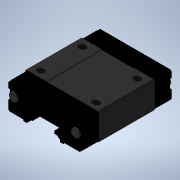
# Autodesk Inventor part: SSEB-MX13_b
Saved by Autodesk Inventor 2021 (Build 250183000, 183)
## iProperties
Created: 2025-02-22
Part Number: SSEB-MX13_b
Material: Generic
Catalog Web Link: www.cadenas.de
Description: SSEB, SSEB-MX, SSEBV, SSEBV-MX, SSE2B, SSE2B-MX, SSE2BV, SSE2BV-MX, SSEBL, SSEBL-MX, SSEBLV, SSEBLV-MX, SSE2BL, SSE2BL-MX, SSE2BLV, SSE2BLV-MX, SEB, SEBV, SE2B, SE2BV, SEBL, SEBLV, SE2BL, SE2BLV_block-Miniature Linear Guides - Short Block, Standard Preload - High/Precision Grade
Vendor: MISUMI
Document SubType Name: Modeling
Designer: psAdmin
Manufacturer: MISUMI
Mass: 6.93419 g
Surface Area: 35.9078 cm^2
Volume: 6.93419 cm^3
Density: 1 g/cm^3
Appearance: PSOLRGB-175-175-175
Category: PARTsolutions
Company: MISUMI
Title: SSEB-MX13
Author: Cadenas PARTsolutions
Comments: Miniature Linear Guides - Short Block, Standard Preload - High/Precision Grade
PSOL_IDENT_0: {$CADENAS_DATA/23d-libs/misumi/metric/06_linear_guides/seb_series/seb_block.prj},367 {VTYP=3D},{NB=S
PSOL_IDENT_1: SEB-MX13_b},{LINA=SSEB-MX13},{NN=SSEB, SSEB-MX, SSEBV, SSEBV-MX, SSE2B, SSE2B-MX, SSE2BV, SSE2BV-MX,
PSOL_IDENT_2: SSEBL, SSEBL-MX, SSEBLV, SSEBLV-MX, SSE2BL, SSE2BL-MX, SSE2BLV, SSE2BLV-MX, SEB, SEBV, SE2B, SE2BV,
PSOL_IDENT_3: SEBL, SEBLV, SE2BL, SE2BLV_block},{DATE=01.06.2021 05:33:03},{GEOMDATE=29.09.2020 01:45:00},{VERSIO
PSOL_IDENT_4: N=},{LINEID=230},{WBVAR=TS,MAT,ST,MX},{WBNUMERIC=}  {NB=SSEB-MX13_b},{LINA=SSEB-MX13},{KT=DUMMY},{PN=
PSOL_IDENT_5: SSEB-MX13},{TS=},{TYPE=SSEB},{H=13},{MAT=S},{ST=S},{ST1='S', 'w/o Surface Treatment','R','Low Temper
PSOL_IDENT_6: ature Black Chrome Plating'},{HARD=56HRC~},{STPN=S},{MX=-MX},{MXALG='', 'w/o MX(Lubrication unit)', '
PSOL_IDENT_7: -MX', 'with MX(Lubrication unit)'},{W=27},{L1=33.9},{B=20},{C=15},{SLL=M3x3.5},{S=3},{LL=3.5},{L2=19
PSOL_IDENT_8: .9},{K=10.0},{CBB=0.5},{W1=12},{W2=7.5},{H1=7.5},{CAA=0.5},{F=25},{G=10.0},{CA1=0.3},{CA2=0.5},{VA1=
PSOL_IDENT_9: 2.3},{HA1=2.0},{WA1=2.5298},{WA2=1.0},{RA1=2.64},{HA2=12.5830},{POIA1=0.1820},{BHA1=22.6},{BHA2=26.5
PSOL_IDENT_10: },{BHA3=26.6},{BHA5=15.0000},{BHA6=26.1},{BHA7=10.8},{BHA8=3.2},{BVA1=4.60},{BVA3=0.30},{BVA4=0.40},
PSOL_IDENT_11: {BVA5=9.50},{BVA6=9.60},{BCA1=0.5},{BCA2H=0.4},{BCA2V=0.25},{BRA1=1.80},{BRA2=1.50},{BDA1=24.00},{BH
PSOL_IDENT_12: B1=14.4600},{BHB2=12.9382},{BVB1=5.6300},{BVB2=2.6106},{BRB1=1.6},{BRB2=1.3000},{BRB3=0.1},{BHC1=5.5
PSOL_IDENT_13: 0},{BHC2=1.0},{BHC3=0.6},{BHC4=0.4},{BHC5=0.5},{MD=6.5}
NB: SSEB-MX13_b
NN: SSEB, SSEB-MX, SSEBV, SSEBV-MX, SSE2B, SSE2B-MX, SSE2BV, SSE2BV-MX, SSEBL, SSEBL-MX, SSEBLV, SSEBLV-MX, SSE2BL, SSE2BL-MX, SSE2BLV, SSE2BLV-MX, SEB, SEBV, SE2B, SE2BV, SEBL, SEBLV, SE2BL, SE2BLV_block
NT: Miniature Linear Guides - Short Block, Standard Preload - High/Precision Grade
NBSYN: $PN._b
LINA: SSEB-MX13
CATALOG: Misumi
PN: SSEB-MX13
TS: Advanced
H: 13
MAT: Stainless Steel
ST: w/o Surface Treatment
MX: with MX(Lubrication unit)
W: 27
L1: 33.9
B: 20
C: 15
SLL: M3x3.5
S: 3
LL: 3.5
L2: 19.9
K: 10
CBB: 0.5
W1: 12
W2: 7.5
H1: 7.5
CAA: 0.5
F: 25
G: 10
CA1: 0.3
CA2: 0.5
VA1: 2.3
HA1: 2
WA1: 2.5298
WA2: 1
RA1: 2.64
HA2: 12.583
POIA1: 0.182
BHA1: 22.6
BHA2: 26.5
BHA3: 26.6
BHA5: 15
BHA6: 26.1
BHA7: 10.8
BHA8: 3.2
BVA1: 4.6
BVA3: 0.3
BVA4: 0.4
BVA5: 9.5
BVA6: 9.6
BCA1: 0.5
BCA2H: 0.4
BCA2V: 0.25
BRA1: 1.8
BRA2: 1.5
BDA1: 24
BHB1: 14.46
BHB2: 12.9382
BVB1: 5.63
BVB2: 2.6106
BRB1: 1.6
BRB2: 1.3
BRB3: 0.1
BHC1: 5.5
BHC2: 1
BHC3: 0.6
BHC4: 0.4
BHC5: 0.5
MD: 6.5
SUPPLIER: MISUMI
ARTICLENO: SSEB-MX13_b
BOMINFO: SSEB-MX13
CREATOR: CADENAS GmbH
Autodesk Inventor part; units mm, degrees
sketch "Sketch_2" plane through (0, 0, 0) normal (0, 0, 1) x (1, 0, 0)
  line L0 (-13.5, 3.5) -> (-13, 3)
  line L1 (-13, 3) -> (-7.5, 3)
  line L2 (-7.5, 3) -> (-7.2754, 3.1)
  line L3 (-7.2754, 3.1) -> (7.2754, 3.1)
  line L4 (7.2754, 3.1) -> (7.5, 3)
  line L5 (7.5, 3) -> (13, 3)
  line L6 (13, 3) -> (13.5, 3.5)
  line L7 (13.5, 3.5) -> (13.5, 12.5)
  line L8 (13.5, 12.5) -> (13, 13)
  line L9 (13, 13) -> (5.8, 13)
  line L10 (5.8, 13) -> (5.4, 12.75)
  line L11 (5.4, 12.75) -> (-5.4, 12.75)
  line L12 (-5.4, 12.75) -> (-5.8, 13)
  line L13 (-5.8, 13) -> (-13, 13)
  line L14 (-13, 13) -> (-13.5, 12.5)
  line L15 (-13.5, 12.5) -> (-13.5, 3.5)
  constraints: 32 end point
extrude "Extrusion1" add sketch "Sketch_2" along normal mid plane 19.9
sketch "Sketch_3" plane through (0, 0, 9.95) normal (0, 0, 1) x (1, 0, 0)
  line L0 (-13.3, 12.2) -> (-13.3, 3.6)
  line L1 (-13.3, 3.6) -> (-12.8, 3.1)
  line L2 (-12.8, 3.1) -> (12.8, 3.1)
  line L3 (12.8, 3.1) -> (13.3, 3.6)
  line L4 (13.3, 3.6) -> (13.3, 12.2)
  line L5 (13.3, 12.2) -> (12.8, 12.7)
  line L6 (12.8, 12.7) -> (-12.8, 12.7)
  line L7 (-12.8, 12.7) -> (-13.3, 12.2)
  constraints: 16 end point
extrude "Extrusion2" add sketch "Sketch_3" along normal blind 7
sketch "Sketch_4" plane through (0, 0, -9.95) normal (0, 0, 1) x (1, 0, 0)
  line L0 (-13.3, 12.2) -> (-13.3, 3.6)
  line L1 (-13.3, 3.6) -> (-12.8, 3.1)
  line L2 (-12.8, 3.1) -> (12.8, 3.1)
  line L3 (12.8, 3.1) -> (13.3, 3.6)
  line L4 (13.3, 3.6) -> (13.3, 12.2)
  line L5 (13.3, 12.2) -> (12.8, 12.7)
  line L6 (12.8, 12.7) -> (-12.8, 12.7)
  line L7 (-12.8, 12.7) -> (-13.3, 12.2)
  constraints: 16 end point
extrude "Extrusion3" add sketch "Sketch_4" against normal blind 7
sketch "Sketch_8" plane through (0, 0, 16.95) normal (0, 0, 1) x (1, 0, 0)
  line L0 (-27, 19.5) -> (-27, 0)
  line L1 (-27, 0) -> (27, 0)
  line L2 (27, 0) -> (27, 19.5)
  line L3 (27, 19.5) -> (-27, 19.5)
  line L4 (-13.25, 12.1) -> (-13.25, 10.2)
  line L5 (-13.25, 10.2) -> (-11.3, 10.2)
  arc A0 (-11.3, 6.6) -> (-11.3, 10.2) centre (-11.3, 8.4) ccw
  line L6 (-11.3, 6.6) -> (-13.25, 6.6)
  line L7 (-13.25, 6.6) -> (-13.25, 3.6)
  line L8 (-13.25, 3.6) -> (-12.75, 3.1)
  line L9 (-12.75, 3.1) -> (12.75, 3.1)
  line L10 (12.75, 3.1) -> (13.25, 3.6)
  line L11 (13.25, 3.6) -> (13.25, 6.6)
  line L12 (13.25, 6.6) -> (11.3, 6.6)
  arc A1 (11.3, 10.2) -> (11.3, 6.6) centre (11.3, 8.4) ccw
  line L13 (11.3, 10.2) -> (13.25, 10.2)
  line L14 (13.25, 10.2) -> (13.25, 12.1)
  line L15 (13.25, 12.1) -> (12.75, 12.6)
  line L16 (12.75, 12.6) -> (-12.75, 12.6)
  line L17 (-12.75, 12.6) -> (-13.25, 12.1)
  constraints: 36 end point, 4 point on circle, 2 centre point
extrude "Extrusion4" cut sketch "Sketch_8" against normal blind 1.5
sketch "Sketch_14" plane through (0, 0, 16.95) normal (0, 0, 1) x (1, 0, 0)
  line L0 (-27, 19.5) -> (-27, 0)
  line L1 (-27, 0) -> (27, 0)
  line L2 (27, 0) -> (27, 19.5)
  line L3 (27, 19.5) -> (-27, 19.5)
  arc A0 (-7.23, 6.5053) -> (-6.4, 5.2932) centre (-5.93, 6.5053) ccw
  arc A1 (-6.4, 5.1068) -> (-6.4, 5.2932) centre (-6.4362, 5.2) ccw
  arc A2 (-6.4, 5.1068) -> (-7.23, 3.8947) centre (-5.93, 3.8947) ccw
  line L4 (-7.23, 3.8947) -> (-7.23, 3.1)
  line L5 (-7.23, 3.1) -> (7.23, 3.1)
  line L6 (7.23, 3.1) -> (7.23, 3.8947)
  arc A3 (7.23, 3.8947) -> (6.4, 5.1068) centre (5.93, 3.8947) ccw
  arc A4 (6.4, 5.2932) -> (6.4, 5.1068) centre (6.4362, 5.2) ccw
  arc A5 (6.4, 5.2932) -> (7.23, 6.5053) centre (5.93, 6.5053) ccw
  line L7 (7.23, 6.5053) -> (7.23, 7.13)
  arc A6 (7.23, 7.13) -> (5.63, 8.73) centre (5.63, 7.13) ccw
  line L8 (5.63, 8.73) -> (-5.63, 8.73)
  arc A7 (-5.63, 8.73) -> (-7.23, 7.13) centre (-5.63, 7.13) ccw
  line L9 (-7.23, 7.13) -> (-7.23, 6.5053)
  constraints: 20 end point, 16 point on circle, 8 centre point
extrude "Extrusion5" cut sketch "Sketch_14" against normal blind 0.5
sketch "Sketch_7" plane through (0, 0, -16.95) normal (0, 0, 1) x (1, 0, 0)
  line L0 (-27, 19.5) -> (-27, 0)
  line L1 (-27, 0) -> (27, 0)
  line L2 (27, 0) -> (27, 19.5)
  line L3 (27, 19.5) -> (-27, 19.5)
  line L4 (-13.25, 12.1) -> (-13.25, 10.2)
  line L5 (-13.25, 10.2) -> (-11.3, 10.2)
  arc A0 (-11.3, 6.6) -> (-11.3, 10.2) centre (-11.3, 8.4) ccw
  line L6 (-11.3, 6.6) -> (-13.25, 6.6)
  line L7 (-13.25, 6.6) -> (-13.25, 3.6)
  line L8 (-13.25, 3.6) -> (-12.75, 3.1)
  line L9 (-12.75, 3.1) -> (12.75, 3.1)
  line L10 (12.75, 3.1) -> (13.25, 3.6)
  line L11 (13.25, 3.6) -> (13.25, 6.6)
  line L12 (13.25, 6.6) -> (11.3, 6.6)
  arc A1 (11.3, 10.2) -> (11.3, 6.6) centre (11.3, 8.4) ccw
  line L13 (11.3, 10.2) -> (13.25, 10.2)
  line L14 (13.25, 10.2) -> (13.25, 12.1)
  line L15 (13.25, 12.1) -> (12.75, 12.6)
  line L16 (12.75, 12.6) -> (-12.75, 12.6)
  line L17 (-12.75, 12.6) -> (-13.25, 12.1)
  constraints: 36 end point, 4 point on circle, 2 centre point
extrude "Extrusion6" cut sketch "Sketch_7" along normal blind 1.5
sketch "Sketch_16" plane through (0, 0, -16.95) normal (0, 0, 1) x (1, 0, 0)
  line L0 (-27, 19.5) -> (-27, 0)
  line L1 (-27, 0) -> (27, 0)
  line L2 (27, 0) -> (27, 19.5)
  line L3 (27, 19.5) -> (-27, 19.5)
  arc A0 (-7.23, 6.5053) -> (-6.4, 5.2932) centre (-5.93, 6.5053) ccw
  arc A1 (-6.4, 5.1068) -> (-6.4, 5.2932) centre (-6.4362, 5.2) ccw
  arc A2 (-6.4, 5.1068) -> (-7.23, 3.8947) centre (-5.93, 3.8947) ccw
  line L4 (-7.23, 3.8947) -> (-7.23, 3.1)
  line L5 (-7.23, 3.1) -> (7.23, 3.1)
  line L6 (7.23, 3.1) -> (7.23, 3.8947)
  arc A3 (7.23, 3.8947) -> (6.4, 5.1068) centre (5.93, 3.8947) ccw
  arc A4 (6.4, 5.2932) -> (6.4, 5.1068) centre (6.4362, 5.2) ccw
  arc A5 (6.4, 5.2932) -> (7.23, 6.5053) centre (5.93, 6.5053) ccw
  line L7 (7.23, 6.5053) -> (7.23, 7.13)
  arc A6 (7.23, 7.13) -> (5.63, 8.73) centre (5.63, 7.13) ccw
  line L8 (5.63, 8.73) -> (-5.63, 8.73)
  arc A7 (-5.63, 8.73) -> (-7.23, 7.13) centre (-5.63, 7.13) ccw
  line L9 (-7.23, 7.13) -> (-7.23, 6.5053)
  constraints: 20 end point, 16 point on circle, 8 centre point
extrude "Extrusion7" cut sketch "Sketch_16" along normal blind 0.5
sketch "Sketch_25" plane through (0, 0, 15.45) normal (0, 0, 1) x (1, 0, 0)
  line L0 (-13.05, 10.2) -> (-13.05, 6.6)
  line L1 (-13.05, 6.6) -> (-11.3, 6.6)
  arc A0 (-11.3, 6.6) -> (-11.3, 10.2) centre (-11.3, 8.4) ccw
  line L2 (-11.3, 10.2) -> (-13.05, 10.2)
  constraints: 6 end point, 2 point on circle, 1 centre point
extrude "Extrusion8" add sketch "Sketch_25" along normal blind 0.6
sketch "Sketch_5" plane through (0, 0, 15.45) normal (0, 0, 1) x (1, 0, 0)
  arc A0 (11.3, 10.2) -> (11.3, 6.6) centre (11.3, 8.4) ccw
  line L0 (11.3, 6.6) -> (13.05, 6.6)
  line L1 (13.05, 6.6) -> (13.05, 10.2)
  line L2 (13.05, 10.2) -> (11.3, 10.2)
  constraints: 6 end point, 2 point on circle, 1 centre point
extrude "Extrusion9" add sketch "Sketch_5" along normal blind 0.6
sketch "Sketch_9" plane through (0, 0, -15.45) normal (0, 0, 1) x (1, 0, 0)
  line L0 (-13.05, 10.2) -> (-13.05, 6.6)
  line L1 (-13.05, 6.6) -> (-11.3, 6.6)
  arc A0 (-11.3, 6.6) -> (-11.3, 10.2) centre (-11.3, 8.4) ccw
  line L2 (-11.3, 10.2) -> (-13.05, 10.2)
  constraints: 6 end point, 2 point on circle, 1 centre point
extrude "Extrusion10" add sketch "Sketch_9" against normal blind 0.6
sketch "Sketch_26" plane through (0, 0, -15.45) normal (0, 0, 1) x (1, 0, 0)
  arc A0 (11.3, 10.2) -> (11.3, 6.6) centre (11.3, 8.4) ccw
  line L0 (11.3, 6.6) -> (13.05, 6.6)
  line L1 (13.05, 6.6) -> (13.05, 10.2)
  line L2 (13.05, 10.2) -> (11.3, 10.2)
  constraints: 6 end point, 2 point on circle, 1 centre point
extrude "Extrusion11" add sketch "Sketch_26" against normal blind 0.6
sketch "Sketch_18" plane through (-11.3, 0, 0) normal (1, 0, 0) x (0, 0, -1)
  line L0 (-16.05, 8.4) -> (-16.65, 8.4)
  line L1 (-16.65, 8.4) -> (-16.65, 9.9)
  line L2 (-16.65, 9.9) -> (-16.05, 9.9)
  line L3 (-16.05, 9.9) -> (-16.05, 8.4)
  line L4 (-16.05, 8.4) -> (-16.65, 8.4)
  constraints: 10 end point
revolve "Revolution1" add sketch "Sketch_18" angle 360 about axis through (-11.3, 8.4, 16.05) along (0, 0, -1)
sketch "Sketch_19" plane through (-11.3, 0, 0) normal (1, 0, 0) x (0, 0, -1)
  line L0 (16.65, 8.4) -> (16.05, 8.4)
  line L1 (16.05, 8.4) -> (16.05, 9.9)
  line L2 (16.05, 9.9) -> (16.65, 9.9)
  line L3 (16.65, 9.9) -> (16.65, 8.4)
  line L4 (16.65, 8.4) -> (16.05, 8.4)
  constraints: 10 end point
revolve "Revolution2" add sketch "Sketch_19" angle 360 about axis through (-11.3, 8.4, -16.65) along (0, 0, -1)
sketch "Sketch_20" plane through (11.3, 0, 0) normal (1, 0, 0) x (0, 0, -1)
  line L0 (-16.05, 8.4) -> (-16.65, 8.4)
  line L1 (-16.65, 8.4) -> (-16.65, 9.9)
  line L2 (-16.65, 9.9) -> (-16.05, 9.9)
  line L3 (-16.05, 9.9) -> (-16.05, 8.4)
  line L4 (-16.05, 8.4) -> (-16.65, 8.4)
  constraints: 10 end point
revolve "Revolution3" add sketch "Sketch_20" angle 360 about axis through (11.3, 8.4, 16.05) along (0, 0, -1)
sketch "Sketch_21" plane through (11.3, 0, 0) normal (1, 0, 0) x (0, 0, -1)
  line L0 (16.65, 8.4) -> (16.05, 8.4)
  line L1 (16.05, 8.4) -> (16.05, 9.9)
  line L2 (16.05, 9.9) -> (16.65, 9.9)
  line L3 (16.65, 9.9) -> (16.65, 8.4)
  line L4 (16.65, 8.4) -> (16.05, 8.4)
  constraints: 10 end point
revolve "Revolution4" add sketch "Sketch_21" angle 360 about axis through (11.3, 8.4, -16.65) along (0, 0, -1)
sketch "Sketch_17" plane through (0, 0, 0) normal (0, 0, 1) x (1, 0, 0)
  line L0 (-6, 7.2) -> (-6, 6.4649)
  line L1 (-6, 6.4649) -> (-5.6315, 6.2522)
  arc A0 (-5.1112, 5.7) -> (-5.6315, 6.2522) centre (-6.2915, 5.109) ccw
  line L2 (-5.1112, 5.7) -> (-4, 5.7)
  line L3 (-4, 5.7) -> (-4, 4.7)
  line L4 (-4, 4.7) -> (-5.1112, 4.7)
  arc A1 (-5.6315, 4.1478) -> (-5.1112, 4.7) centre (-6.2915, 5.291) ccw
  line L5 (-5.6315, 4.1478) -> (-6, 3.9351)
  line L6 (-6, 3.9351) -> (-6, 0.5)
  line L7 (-6, 0.5) -> (-5.5, 0)
  line L8 (-5.5, 0) -> (5.5, 0)
  line L9 (5.5, 0) -> (6, 0.5)
  line L10 (6, 0.5) -> (6, 3.9351)
  line L11 (6, 3.9351) -> (5.6315, 4.1478)
  arc A2 (5.1112, 4.7) -> (5.6315, 4.1478) centre (6.2915, 5.291) ccw
  line L12 (5.1112, 4.7) -> (4, 4.7)
  line L13 (4, 4.7) -> (4, 5.7)
  line L14 (4, 5.7) -> (5.1112, 5.7)
  arc A3 (5.6315, 6.2522) -> (5.1112, 5.7) centre (6.2915, 5.109) ccw
  line L15 (5.6315, 6.2522) -> (6, 6.4649)
  line L16 (6, 6.4649) -> (6, 7.2)
  line L17 (6, 7.2) -> (5.7, 7.5)
  line L18 (5.7, 7.5) -> (-5.7, 7.5)
  line L19 (-5.7, 7.5) -> (-6, 7.2)
  constraints: 40 end point, 8 point on circle, 4 centre point
extrude "Extrusion12" cut sketch "Sketch_17" along normal mid plane 19.9
sketch "Sketch_11" plane through (0, 0, 9.95) normal (0, 0, 1) x (1, 0, 0)
  line L0 (-6, 7.2) -> (-6, 6.4649)
  line L1 (-6, 6.4649) -> (-5.6315, 6.2522)
  arc A0 (-5.1112, 5.7) -> (-5.6315, 6.2522) centre (-6.2915, 5.109) ccw
  line L2 (-5.1112, 5.7) -> (-4, 5.7)
  line L3 (-4, 5.7) -> (-4, 4.7)
  line L4 (-4, 4.7) -> (-5.1112, 4.7)
  arc A1 (-5.6315, 4.1478) -> (-5.1112, 4.7) centre (-6.2915, 5.291) ccw
  line L5 (-5.6315, 4.1478) -> (-6, 3.9351)
  line L6 (-6, 3.9351) -> (-6, 0.5)
  line L7 (-6, 0.5) -> (-5.5, 0)
  line L8 (-5.5, 0) -> (5.5, 0)
  line L9 (5.5, 0) -> (6, 0.5)
  line L10 (6, 0.5) -> (6, 3.9351)
  line L11 (6, 3.9351) -> (5.6315, 4.1478)
  arc A2 (5.1112, 4.7) -> (5.6315, 4.1478) centre (6.2915, 5.291) ccw
  line L12 (5.1112, 4.7) -> (4, 4.7)
  line L13 (4, 4.7) -> (4, 5.7)
  line L14 (4, 5.7) -> (5.1112, 5.7)
  arc A3 (5.6315, 6.2522) -> (5.1112, 5.7) centre (6.2915, 5.109) ccw
  line L15 (5.6315, 6.2522) -> (6, 6.4649)
  line L16 (6, 6.4649) -> (6, 7.2)
  line L17 (6, 7.2) -> (5.7, 7.5)
  line L18 (5.7, 7.5) -> (-5.7, 7.5)
  line L19 (-5.7, 7.5) -> (-6, 7.2)
  constraints: 40 end point, 8 point on circle, 4 centre point
extrude "Extrusion13" cut sketch "Sketch_11" along normal blind 9.95
sketch "Sketch_22" plane through (0, 0, 9.95) normal (0, 0, 1) x (1, 0, 0)
  line L0 (-27, 19.5) -> (-27, 0)
  line L1 (-27, 0) -> (27, 0)
  line L2 (27, 0) -> (27, 19.5)
  line L3 (27, 19.5) -> (-27, 19.5)
  line L4 (-13.3, 12.25) -> (-13.3, 3.6)
  line L5 (-13.3, 3.6) -> (-12.85, 3.15)
  line L6 (-12.85, 3.15) -> (-6.05, 3.15)
  line L7 (-6.05, 3.15) -> (-6.05, 3.9851)
  line L8 (-6.05, 3.9851) -> (-5.7055, 4.1643)
  arc A0 (-5.7055, 4.1643) -> (-5.1425, 4.75) centre (-6.2915, 5.291) ccw
  line L9 (-5.1425, 4.75) -> (-4.05, 4.75)
  line L10 (-4.05, 4.75) -> (-4.05, 5.65)
  line L11 (-4.05, 5.65) -> (-5.1425, 5.65)
  arc A1 (-5.1425, 5.65) -> (-5.7055, 6.2357) centre (-6.2915, 5.109) ccw
  line L12 (-5.7055, 6.2357) -> (-6.05, 6.4149)
  line L13 (-6.05, 6.4149) -> (-6.05, 7.25)
  line L14 (-6.05, 7.25) -> (-5.75, 7.55)
  line L15 (-5.75, 7.55) -> (5.75, 7.55)
  line L16 (5.75, 7.55) -> (6.05, 7.25)
  line L17 (6.05, 7.25) -> (6.05, 6.4149)
  line L18 (6.05, 6.4149) -> (5.7055, 6.2357)
  arc A2 (5.7055, 6.2357) -> (5.1425, 5.65) centre (6.2915, 5.109) ccw
  line L19 (5.1425, 5.65) -> (4.05, 5.65)
  line L20 (4.05, 5.65) -> (4.05, 4.75)
  line L21 (4.05, 4.75) -> (5.1425, 4.75)
  arc A3 (5.1425, 4.75) -> (5.7055, 4.1643) centre (6.2915, 5.291) ccw
  line L22 (5.7055, 4.1643) -> (6.05, 3.9851)
  line L23 (6.05, 3.9851) -> (6.05, 3.15)
  line L24 (6.05, 3.15) -> (12.85, 3.15)
  line L25 (12.85, 3.15) -> (13.3, 3.6)
  line L26 (13.3, 3.6) -> (13.3, 12.25)
  line L27 (13.3, 12.25) -> (12.85, 12.7)
  line L28 (12.85, 12.7) -> (-12.85, 12.7)
  line L29 (-12.85, 12.7) -> (-13.3, 12.25)
  constraints: 60 end point, 8 point on circle, 4 centre point
extrude "Extrusion14" cut sketch "Sketch_22" along normal blind 0.05
sketch "Sketch_10" plane through (0, 0, -9.95) normal (0, 0, 1) x (1, 0, 0)
  line L0 (-6, 7.2) -> (-6, 6.4649)
  line L1 (-6, 6.4649) -> (-5.6315, 6.2522)
  arc A0 (-5.1112, 5.7) -> (-5.6315, 6.2522) centre (-6.2915, 5.109) ccw
  line L2 (-5.1112, 5.7) -> (-4, 5.7)
  line L3 (-4, 5.7) -> (-4, 4.7)
  line L4 (-4, 4.7) -> (-5.1112, 4.7)
  arc A1 (-5.6315, 4.1478) -> (-5.1112, 4.7) centre (-6.2915, 5.291) ccw
  line L5 (-5.6315, 4.1478) -> (-6, 3.9351)
  line L6 (-6, 3.9351) -> (-6, 0.5)
  line L7 (-6, 0.5) -> (-5.5, 0)
  line L8 (-5.5, 0) -> (5.5, 0)
  line L9 (5.5, 0) -> (6, 0.5)
  line L10 (6, 0.5) -> (6, 3.9351)
  line L11 (6, 3.9351) -> (5.6315, 4.1478)
  arc A2 (5.1112, 4.7) -> (5.6315, 4.1478) centre (6.2915, 5.291) ccw
  line L12 (5.1112, 4.7) -> (4, 4.7)
  line L13 (4, 4.7) -> (4, 5.7)
  line L14 (4, 5.7) -> (5.1112, 5.7)
  arc A3 (5.6315, 6.2522) -> (5.1112, 5.7) centre (6.2915, 5.109) ccw
  line L15 (5.6315, 6.2522) -> (6, 6.4649)
  line L16 (6, 6.4649) -> (6, 7.2)
  line L17 (6, 7.2) -> (5.7, 7.5)
  line L18 (5.7, 7.5) -> (-5.7, 7.5)
  line L19 (-5.7, 7.5) -> (-6, 7.2)
  constraints: 40 end point, 8 point on circle, 4 centre point
extrude "Extrusion15" cut sketch "Sketch_10" against normal blind 9.95
sketch "Sketch_23" plane through (0, 0, -9.95) normal (0, 0, 1) x (1, 0, 0)
  line L0 (-27, 19.5) -> (-27, 0)
  line L1 (-27, 0) -> (27, 0)
  line L2 (27, 0) -> (27, 19.5)
  line L3 (27, 19.5) -> (-27, 19.5)
  line L4 (-13.3, 12.25) -> (-13.3, 3.6)
  line L5 (-13.3, 3.6) -> (-12.85, 3.15)
  line L6 (-12.85, 3.15) -> (-6.05, 3.15)
  line L7 (-6.05, 3.15) -> (-6.05, 3.9851)
  line L8 (-6.05, 3.9851) -> (-5.7055, 4.1643)
  arc A0 (-5.7055, 4.1643) -> (-5.1425, 4.75) centre (-6.2915, 5.291) ccw
  line L9 (-5.1425, 4.75) -> (-4.05, 4.75)
  line L10 (-4.05, 4.75) -> (-4.05, 5.65)
  line L11 (-4.05, 5.65) -> (-5.1425, 5.65)
  arc A1 (-5.1425, 5.65) -> (-5.7055, 6.2357) centre (-6.2915, 5.109) ccw
  line L12 (-5.7055, 6.2357) -> (-6.05, 6.4149)
  line L13 (-6.05, 6.4149) -> (-6.05, 7.25)
  line L14 (-6.05, 7.25) -> (-5.75, 7.55)
  line L15 (-5.75, 7.55) -> (5.75, 7.55)
  line L16 (5.75, 7.55) -> (6.05, 7.25)
  line L17 (6.05, 7.25) -> (6.05, 6.4149)
  line L18 (6.05, 6.4149) -> (5.7055, 6.2357)
  arc A2 (5.7055, 6.2357) -> (5.1425, 5.65) centre (6.2915, 5.109) ccw
  line L19 (5.1425, 5.65) -> (4.05, 5.65)
  line L20 (4.05, 5.65) -> (4.05, 4.75)
  line L21 (4.05, 4.75) -> (5.1425, 4.75)
  arc A3 (5.1425, 4.75) -> (5.7055, 4.1643) centre (6.2915, 5.291) ccw
  line L22 (5.7055, 4.1643) -> (6.05, 3.9851)
  line L23 (6.05, 3.9851) -> (6.05, 3.15)
  line L24 (6.05, 3.15) -> (12.85, 3.15)
  line L25 (12.85, 3.15) -> (13.3, 3.6)
  line L26 (13.3, 3.6) -> (13.3, 12.25)
  line L27 (13.3, 12.25) -> (12.85, 12.7)
  line L28 (12.85, 12.7) -> (-12.85, 12.7)
  line L29 (-12.85, 12.7) -> (-13.3, 12.25)
  constraints: 60 end point, 8 point on circle, 4 centre point
extrude "Extrusion16" cut sketch "Sketch_23" against normal blind 0.05
sketch "Sketch21" plane through (-13, 13, 9.95) normal (0, 1, 0) x (1, 0, 0)
  point P0 (3, 17.45)
hole "Hole1" at (-10, 13, -7.5) direction (0, -1, 0) diameter 2.459 depth 6.5 tip angle 120 countersink diameter 3 countersink angle 90 thread size "M3x0.5" class "6H" standard "ISO Metric profile"
pattern_linear "Rectangular Pattern1" count 2 spacing 20 along (1, 0, 0) count 2 spacing 15 along (0, 0, 1) of "Hole1"
ref_plane "to_rail_XY" through (0, 7.5, 0) normal (0, 0, 1) x (1, 0, 0)
ref_plane "to_rail_YZ" through (0, 7.5, 0) normal (1, 0, 0) x (0, 1, 0)
ref_plane "to_rail_ZX" through (0, 7.5, 0) normal (0, 1, 0) x (0, 0, 1)
body "Solid1"
